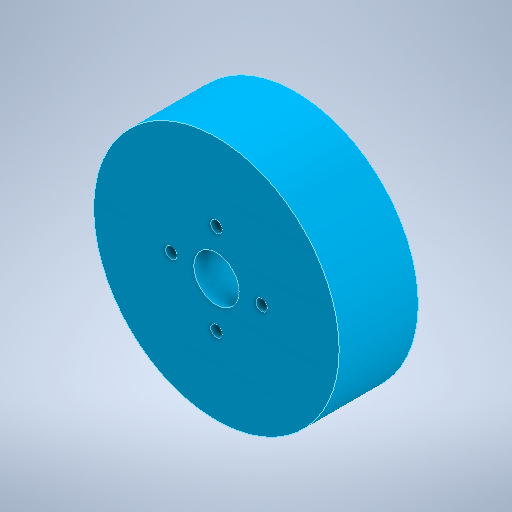
# Autodesk Inventor part: small_tire
Saved by Autodesk Inventor 2025.1 (Build 291241000, 241)
## iProperties
Created: 2024-12-20
Part Number: small_tire
Material: ゴム、シリコーン
Document SubType Name: Modeling
Designer: yuki0520
Density: 1.25 g/cm^3
Appearance: スカイ ブルー 標準
Author: yuki0520
Autodesk Inventor part; units mm, degrees
ref_plane "YZ Plane" through (0, 0, 0) normal (1, 0, 0) x (0, 1, 0)
ref_plane "XZ Plane" through (0, 0, 0) normal (0, 1, 0) x (-1, 0, 0)
ref_plane "XY Plane" through (0, 0, 0) normal (0, 0, 1) x (1, 0, 0)
sketch "スケッチ1" plane through (0, 0, 0) normal (0, 0, 1) x (1, 0, 0)
  circle A0 centre (0, 0) radius 7
  circle A1 centre (0, 0) radius 38
  dimension "d0" = 14
  dimension "d1" = 76
  constraints: 2 centre point, 2 coincident
  measures "d0" diameter of A0
  measures "d1" diameter of A1
extrude "押し出し1" add sketch "スケッチ1" along normal blind 24.5
sketch "スケッチ2" plane through (0, 0, 24.5) normal (0, 0, 1) x (1, 0, 0)
  circle A0 centre (0, 0) radius 7 projected
  circle A1 centre (0, 0) radius 14
  point P0 (0, 14)
  point P1 (-14, 0)
  point P2 (0, -14)
  point P3 (14, 0)
  dimension "d4" = 28
  dimension "d7" = 360
  constraints: 1 coincident, 1 vertical alignment, 7 other
hole "穴1" at (0, 14, 24.5) at (-14, 0, 24.5) at (0, -14, 24.5) at (14, 0, 24.5) direction (0, 0, -1) diameter 3.5 end through all
